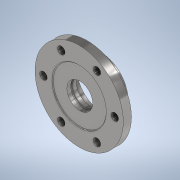
# Autodesk Inventor part: 轴承端盖1
Saved by Autodesk Inventor 2020 (Build 240168000, 168)
## iProperties
Created: 2021-06-16
Part Number: 轴承端盖1
Material: 常规
Document SubType Name: Modeling
Designer: dell
Density: 1 g/cm^3
Appearance: 默认
Author: dell
Autodesk Inventor part; units mm, degrees
ref_plane "工作平面1" through (0, 0, 0) normal (0, 0, 1) x (1, 0, 0)
sketch "草图1" plane through (0, 0, 0) normal (0, 0, 1) x (1, 0, 0)
  arc A0 (-32.5, -65) -> (-32.5, 65) centre (-32.5, 0) ccw construction
  line L0 (-32.5, 40) -> (-32.5, 65) construction
  arc A1 (-32.5, -40) -> (-32.5, 40) centre (-32.5, 0) ccw construction
  line L1 (-32.5, -65) -> (-32.5, -40) construction
  circle A2 centre (-32.5, 0) radius 65
  circle A3 centre (-32.5, 0) radius 40
  circle A4 centre (-32.5, 0) radius 52.5 construction
  circle A5 centre (-85, 0) radius 5.5
  line L2 (-123.5, 0) -> (58.5, 0) construction
  circle A6 centre (-58.75, -45.4663) radius 5.5
  circle A7 centre (-6.25, -45.4663) radius 5.5
  circle A8 centre (20, 0) radius 5.5
  circle A9 centre (-6.25, 45.4663) radius 5.5
  circle A10 centre (-58.75, 45.4663) radius 5.5
  circle A11 centre (-32.5, 0) radius 35
  point P0 (0, 0)
  dimension "d0" = 105
  dimension "d1" = 11
  dimension "d4" = 360
  dimension "d6" = 70
  constraints: 10 centre point, 5 coincident, 2 concentric, 2 point on circle, 1 point on line, 13 other
  measures "d0" diameter of A4
  measures "d1" diameter of A5
  measures "d6" diameter of A11
extrude "拉伸1" add sketch "草图1" along normal blind 12 contours A2 | A3 | A11
sketch "草图2" plane through (-32.5, 0, 0) normal (0, 0, -1) x (-1, 0, 0)
  circle A0 centre (0, 0) radius 65 construction
  circle A1 centre (0, 0) radius 35
  circle A2 centre (0, 0) radius 40
  point P0 (-32.5, 0)
  dimension "d9" = 70
  dimension "d10" = 80
  constraints: 2 centre point, 2 coincident
  measures "d9" diameter of A1
  measures "d10" diameter of A2
extrude "拉伸2" add sketch "草图2" along normal blind 20
sketch "草图3" plane through (-32.5, 0, 12) normal (0, 0, 1) x (1, 0, 0)
  circle A0 centre (0, 0) radius 18 construction
  circle A1 centre (0, 0) radius 19
  point P0 (32.5, 0)
  dimension "d23" = 38
  constraints: 1 centre point
  measures "d23" diameter of A1
extrude "拉伸3" cut sketch "草图3" against normal up to surface (12 mm away)
sketch "草图4" plane through (-32.5, 0, 12) normal (0, 0, 1) x (1, 0, 0)
  line L0 (-91, 0) -> (91, 0) construction
  circle A0 centre (0, 0) radius 65 construction
  line L1 (0, -101.0835) -> (0, 92.1895) construction
  circle A1 centre (0, 0) radius 40
  circle A2 centre (-52.5, 0) radius 5.5 construction
  circle A3 centre (0, 0) radius 19 projected
  point P0 (32.5, 0)
  dimension "d16" = 80
  constraints: 2 end point, 1 centre point, 1 coincident, 1 point on line, 1 vertical
  measures "d16" diameter of A1
extrude "拉伸4" cut sketch "草图4" against normal blind 1
fillet "圆角1" radius 1 1 edges at (-72.5, 0, 11)
ref_plane "工作平面2" through (-32.5, 0, 6) normal (0, 0, 1) x (1, 0, 0)
sketch "草图5" plane through (-32.5, 0, 0) normal (0, 0, -1) x (-1, 0, 0)
  circle A0 centre (0, 0) radius 40 projected
  circle A1 centre (0, 0) radius 39
  point P0 (-32.5, 0)
  dimension "d20" = 1
  constraints: 1 centre point
  measures "d20" radial gap between concentric circles of A0 A1
extrude "拉伸5" cut sketch "草图5" along normal blind 2
sketch "草图6" plane through (-32.5, 0, 0) normal (0, 0, -1) x (-1, 0, 0)
  circle A0 centre (0, 0) radius 19 projected
  circle A1 centre (0, 0) radius 35 projected
  point P0 (-32.5, 0)
extrude "拉伸6" add sketch "草图6" along normal blind 3
ref_plane "工作平面3" through (-32.5, 0, 4) normal (0, 0, 1) x (1, 0, 0)
sketch "草图7" plane through (-32.5, 0, 4) normal (0, 0, 1) x (1, 0, 0)
  circle A0 centre (0, 0) radius 19 construction
  circle A1 centre (0, 0) radius 20.4
  point P0 (32.5, 0)
  dimension "d27" = 40.8
  constraints: 1 centre point, 1 coincident
  measures "d27" diameter of A1
extrude "拉伸7" cut sketch "草图7" against normal mid plane 2.65
